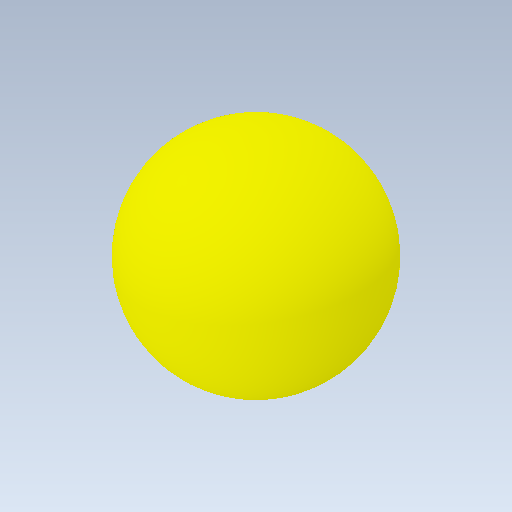
# Autodesk Inventor part: SKF_608_PART3
Saved by Autodesk Inventor 2021 (Build 250183000, 183)
## iProperties
Created: 2022-07-09
Part Number: SKF_608_PART3
Material: Stahl
Catalog Web Link: www.cadenas.de
Description: -Deep groove ball bearings
Vendor: SKF
Document SubType Name: Modeling
Designer: psAdmin
Manufacturer: SKF
Mass: 12 g
Surface Area: 0.494894 cm^2
Volume: 0.0327372 cm^3
Density: 7.85 g/cm^3
Appearance: Platte
Category: PARTsolutions
Company: SKF
PSOL_IDENT_0: {$CADENAS_DATA/23d-libs/skf/bearings_units_and_housings/ball_bearings/deep_groove_ball_bearings/bb1_
PSOL_IDENT_1: 001_101.prj},192 {VTYP=3D},{NB=SKF_608_PART3},{LINA=SKF_608_PART3},{NN=BB1_001_101_PART3},{NOPRJ=TRU
PSOL_IDENT_2: E},{DATE=08.07.2022 10:24:27},{GEOMDATE=04.07.2022 10:54:51},{VERSION=},{LINEID=7910},{WBVAR=},{WBNU
PSOL_IDENT_3: MERIC=}  {NB=SKF_608_PART3},{LINA=SKF_608_PART3},{KT=DUMMY},{DESIGNATION=608},{R12=0.30},{DD=8.000},
PSOL_IDENT_4: {D=22.000},{B=7.000},{C=},{CX=},{CXX=},{CA=0.000},{XXVARIANT=},{XXDESIGN=Single row},{XXSEALING=No s
PSOL_IDENT_5: eals},{DESIGN=dgbb1},{DESIGNIR=dgbb1},{VARIANT=},{DD1=12.15},{DD2=},{DD2X=},{DD2A=0.00},{D1=17.60},{
PSOL_IDENT_6: D1X=0.00},{D2=19.2},{D2A=19.20},{D3=},{D3X=},{D3A=0.000},{D4=},{HH=0.000},{BB=0.000},{BBX=},{BBA=0.0
PSOL_IDENT_7: 00},{FF=},{R0MAX=0.000},{R0=0.000},{PITCH=14.70},{DW=3.969},{DDAMIN=10.000},{DDAMAX=0.000},{DDBMIN=0
PSOL_IDENT_8: .000},{DDBMAX=0.000},{DBMIN=0.000},{DAMAX=20.000},{BBAMIN=0.000},{CAMAX=0.000},{RAMAX=0.300},{LOAD1=
PSOL_IDENT_9: 3.450},{LOAD2=1.370},{LOAD3=0.057},{SPEED1=75000},{SPEED2=48000},{KR=0.025},{F0=12.000},{Z=7},{II=1}
PSOL_IDENT_10: ,{MASS=0.012},{BEARING=608},{RING=},{HELP=2.200},{HELP2=1.400},{DD1ALG=6.075},{YALG=6.075},{PITCH1=1
PSOL_IDENT_11: 4.700},{DW1=3.969},{YALG1=8.800},{HALG1=2.200},{SH=6.075},{CU=0.606},{HALG=2.075},{B1=0},{SHIELDHELP=
PSOL_IDENT_12: 1},{D4A=0.000},{FFA=0.000},{RS1=},{HELP3=0}
NB: SKF_608_PART3
NT: Deep groove ball bearings
NBSYN: SKF_$DESIGNATION._PART3
LINA: SKF_608_PART3
CATALOG: SKF
DESIGNATION: 608
R12: 0.3
DD: 8
D: 22
B: 7
XXDESIGN: Single row
XXSEALING: No seals
D2: 19.2
LOAD1: 3.45
LOAD2: 1.37
LOAD3: 0.057
SPEED1: 75000
SPEED2: 48000
BEARING: 608
SUPPLIER: SKF
ARTICLENO: SKF_608_PART3
BOMINFO: SKF_608_PART3
CREATOR: CADENAS GmbH
Title: SKF_608_PART3
Author: Cadenas PARTsolutions
Comments: Deep groove ball bearings
Autodesk Inventor part; units mm, degrees
ref_plane "YZ Plane" through (0, 0, 0) normal (1, 0, 0) x (0, 1, 0)
ref_plane "XZ Plane" through (0, 0, 0) normal (0, 1, 0) x (-1, 0, 0)
ref_plane "XY Plane" through (0, 0, 0) normal (0, 0, 1) x (1, 0, 0)
sketch "Sketch_6" plane through (0, 0, 0) normal (0, 0, 1) x (1, 0, 0)
  line L0 (5.4845, 7.35) -> (1.5155, 7.35)
  arc A0 (5.4845, 7.35) -> (1.5155, 7.35) centre (3.5, 7.35) ccw
  line L1 (5.4845, 7.35) -> (1.5155, 7.35)
  dimension "d0" = 360
  constraints: 4 end point, 2 point on circle, 1 centre point
revolve "Revolution1" add sketch "Sketch_6" angle 360 about axis through (5.4845, 7.35, 0) along (1, 0, 0)
body "Solid1"
